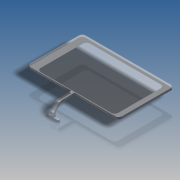
# Autodesk Inventor part: 99148p01-TransClear
Saved by Autodesk Inventor 2016 SP2 (Build 200236200, 236)
## iProperties
Created: 2015-08-19
Part Number: 99148p01-TransClear
Material: Polycarbonate
Document SubType Name: Modeling
Designer: D. Kohfeld
Mass: 2.38771 g
Surface Area: 43.6818 cm^2
Volume: 1.98976 cm^3
Density: 1.2 g/cm^3
Appearance: TransClear
Author: D. Kohfeld
Autodesk Inventor part; units mm, degrees
ref_plane "YZ Plane" through (0, 0, 0) normal (1, 0, 0) x (0, 1, 0)
ref_plane "XZ Plane" through (0, 0, 0) normal (0, 1, 0) x (-1, 0, 0)
ref_plane "XY Plane" through (0, 0, 0) normal (0, 0, 1) x (1, 0, 0)
sketch "Sketch2" plane through (0, 0, 0) normal (0, 1, 0) x (-1, 0, 0)
  line L0 (-24, 15.6) -> (24, 15.6)
  line L1 (26, 13.6) -> (26, -13.6)
  line L2 (24, -15.6) -> (-24, -15.6)
  line L3 (-26, -13.6) -> (-26, 13.6)
  arc A0 (-24, 15.6) -> (-26, 13.6) centre (-24, 13.6) ccw
  arc A1 (-26, -13.6) -> (-24, -15.6) centre (-24, -13.6) ccw
  arc A2 (24, -15.6) -> (26, -13.6) centre (24, -13.6) ccw
  arc A3 (26, 13.6) -> (24, 15.6) centre (24, 13.6) ccw
  line L4 (20, 14) -> (-20, 14)
  line L5 (-22, 12) -> (-22, -12)
  line L6 (-20, -14) -> (20, -14)
  line L7 (22, -12) -> (22, 12)
  arc A4 (22, 12) -> (20, 14) centre (20, 12) ccw
  arc A5 (-20, 14) -> (-22, 12) centre (-20, 12) ccw
  arc A6 (-22, -12) -> (-20, -14) centre (-20, -12) ccw
  arc A7 (20, -14) -> (22, -12) centre (20, -12) ccw
  line L8 (-1, 15.6) -> (-1, 23.6)
  line L9 (-1, 23.6) -> (1, 23.6)
  line L10 (1, 23.6) -> (1, 15.6)
  point P0 (0, 0)
  point P1 (26, -15.6)
  point P2 (-26, -15.6)
  point P3 (0, 15.6)
  point P4 (-26, 0)
  point P5 (0, 14)
  point P6 (-22, 0)
  point P7 (0, 23.6)
  dimension "d0" = 31.2
  dimension "d1" = 52
  dimension "d2" = 2
  dimension "d3" = 28
  dimension "d4" = 44
  dimension "d5" = 2
  dimension "d22" = 2
  dimension "d23" = 8
  constraints: 22 end point, 16 point on circle, 16 tangent, 8 centre point, 6 equal radius, 6 point on line, 5 midpoint, 4 parallel, 3 horizontal, 3 vertical alignment, 2 horizontal alignment, 2 perpendicular, 2 vertical
  measures "d0" distance between parallel lines of L0 L2
  measures "d1" distance of point (26, -15.6) point (-26, -15.6)
  measures "d2" radius of A0
  measures "d3" distance between parallel lines of L6 L4
  measures "d4" distance between parallel lines of L5 L7
  measures "d5" radius of A4
  measures "d22" distance between parallel lines of L8 L10
  measures "d23" distance between parallel lines of L0 L9
extrude "Extrusion1" add sketch "Sketch2" along normal blind 1.2 contours L0 A3 L1 A2 L2 A1 L3 A0 | A4 L7 A7 L6 A6 L5 A5 L4
sketch "Sketch3" plane through (0, 0, 0) normal (1, 0, 0) x (0, 1, 0)
  line L0 (0, 15.6) -> (1.2, 15.6) projected
  arc A0 (1.2, 22.4) -> (0.0065, 25.0774) centre (-2.4, 22.4) ccw
  line L1 (0.0065, 25.0774) -> (-2.8, 27.6)
  line L2 (-2.8, 27.6) -> (-5.2, 27.6)
  line L3 (-5.2, 27.6) -> (-5.2, 26.4)
  line L4 (-5.2, 26.4) -> (-2.8, 26.4)
  line L5 (-2.8, 26.4) -> (0, 23.6)
  line L6 (0, 23.6) -> (0, 15.6)
  line L7 (-5.2, 27.6) -> (-6.8, 27.6)
  line L8 (-6.8, 27.6) -> (-6.8, 26.4)
  line L9 (-6.8, 26.4) -> (-5.2, 26.4)
  line L10 (1.2, 22.4) -> (1.2, 15.6)
  point P0 (0, 0)
  dimension "d10" = 6.8
  dimension "d11" = 4
  dimension "d12" = 1.2
  dimension "d13" = 1.6
  dimension "d14" = 12
  dimension "d15" = 8
  dimension "d16" = 6.8
  dimension "d17" = 3.6
  constraints: 20 end point, 4 horizontal, 4 vertical, 2 point on circle, 2 tangent, 1 centre point, 1 vertical alignment
  measures "d10" distance between parallel lines of L8 L6
  measures "d11" distance from line of L1.end L8
  measures "d12" distance between parallel lines of L9 L7
  measures "d13" distance between parallel lines of L8 L3
  measures "d14" distance between parallel lines of L2 L0
  measures "d15" distance from line of L5.end L0
  measures "d16" distance from line of A0.centre L0
  measures "d17" radius of A0
extrude "Extrusion3" add sketch "Sketch3" along normal mid plane 2 contours L6 L5 L4 L3 L2 L1 A0 L10 L0
extrude "Extrusion4" add sketch "Sketch3" along normal mid plane 6.8 contours L9 L8 L7 L3
extrude "Extrusion2" add sketch "Sketch2" against normal blind 0.001 separate body
fillet "Fillet1" radius 0.1 38 edges at (-25.4142, 1.2, 15.0142) (-26, 1.2, 0) (-25.4142, 1.2, -15.0142) (0, 1.2, -15.6) (25.4142, 1.2, -15.0142) (26, 1.2, 0) (25.4142, 1.2, 15.0142) (12.5, 1.2, 15.6) (-12.5, 1.2, 15.6) (-1, 1.2, 19) (-1, -1.3967, 26.3387) (-1, 0.8881, 23.8657) (1, -1.3967, 26.3387) (1, 1.2, 19) (1, 0.8881, 23.8657) (0, -2.8, 27.6) (1, -1.4, 25) (-1, -1.4, 25) (1, -4, 26.4) (1, -4, 27.6) (-1, -4, 27.6) (-1, -4, 26.4) (-2.2, -5.2, 26.4) (-3.4, -5.2, 27) (-2.2, -5.2, 27.6) (-3.4, -6, 27.6) (-3.4, -6, 26.4) (-3.4, -6.8, 27) (0, -6.8, 27.6) (0, -6.8, 26.4) (2.2, -5.2, 27.6) (2.2, -5.2, 26.4) (3.4, -5.2, 27) (3.4, -6, 26.4) (3.4, -6, 27.6) (3.4, -6.8, 27) (1, -0.0005, 23.6) (-1, -0.0005, 23.6)
equation "\"d23\" = lu"
equation "\"d13\" = wall"
equation "\"d15\" = lu"
equation "\"lu\" = 8"
equation "\"wall\" = 1.6"
